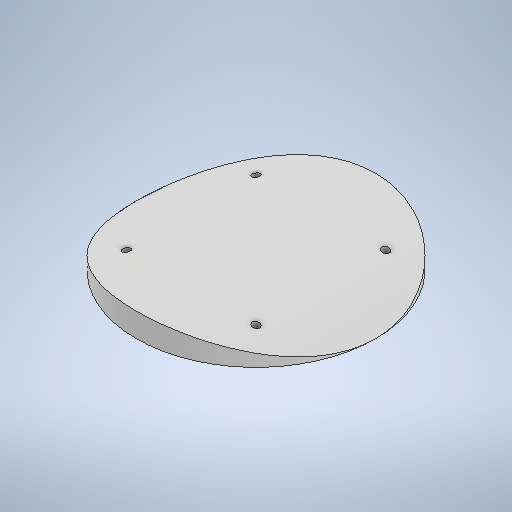
# Autodesk Inventor part: TopHead
Saved by Autodesk Inventor 2025 (Build 290162000, 162)
## iProperties
Created: 2025-09-02
Part Number: TopHead
Material: Generic
Document SubType Name: Modeling
Designer: wangb
Density: 1 g/cm^3
Appearance: Default
Author: wangb
Autodesk Inventor part; units mm, degrees
ref_plane "YZ Plane" through (0, 0, 0) normal (1, 0, 0) x (0, 1, 0)
ref_plane "XZ Plane" through (0, 0, 0) normal (0, 1, 0) x (-1, 0, 0)
ref_plane "XY Plane" through (0, 0, 0) normal (0, 0, 1) x (1, 0, 0)
sketch "Sketch1" plane through (0, 0, 0) normal (0, 0, 1) x (1, 0, 0)
  arc A0 (76.5789, 0) -> (-8.4211, 0) centre (34.0789, -102.0754) ccw
  line L0 (-8.4211, 0) -> (76.5789, 0)
  point P0 (0, 0)
  dimension "d0" = 85
  constraints: 2 end point, 2 point on circle, 1 centre point, 1 horizontal
  measures "d0" distance of L0.start L0.end
extrude "Extrusion1" add sketch "Sketch1" along normal blind 85
sketch "Sketch2" plane through (-8.4211, 0, 0) normal (0, -1, 0) x (1, 0, 0)
  circle A0 centre (7.5, 77.5) radius 0.75
  circle A1 centre (7.5, 7.5) radius 0.75
  circle A2 centre (77.5, 77.5) radius 0.75
  circle A3 centre (77.5, 7.5) radius 0.75
  line L0 (0, 85) -> (85, 85) projected
  line L1 (0, 0) -> (85, 0) projected
  line L2 (85, 0) -> (85, 85) projected
  point P0 (8.4211, 0)
  point P1 (36.7967, 13.095)
  dimension "d3" = 1.5
  dimension "d4" = 1.5
  dimension "d5" = 1.5
  dimension "d6" = 1.5
  dimension "d7" = 70
  dimension "d8" = 7.5
  dimension "d9" = 7.5
  dimension "d10" = 70
  dimension "d11" = 70
  dimension "d12" = 70
  dimension "d13" = 7.5
  dimension "d14" = 7.5
  constraints: 4 centre point
  measures "d3" diameter of A0
  measures "d4" diameter of A1
  measures "d5" diameter of A2
  measures "d6" diameter of A3
  measures "d7" distance of A1.centre A0.centre
  measures "d8" distance from line of L0 A0.centre
  measures "d9" distance from line of L1 A1.centre
  measures "d10" distance of A0.centre A2.centre
  measures "d11" distance of A1.centre A3.centre
  measures "d12" distance of A3.centre A2.centre
  measures "d13" distance from line of L1 A3.centre
  measures "d14" distance from line of L2 A2.centre
extrude "Extrusion2" cut sketch "Sketch2" against normal blind 85
sketch "Sketch3" plane through (-8.4211, 0, 0) normal (0, -1, 0) x (1, 0, 0)
  line L0 (0, 0) -> (0, 85) projected
  line L1 (0, 42.5) -> (85, 42.5)
  line L2 (85, 0) -> (85, 85) projected
  line L3 (0, 85) -> (85, 85) projected
  line L4 (42.5, 85) -> (42.5, 0)
  circle A0 centre (42.5, 42.5) radius 42.5
  line L5 (0, 0) -> (85, 0) projected
  line L6 (85, 85) -> (0, 85)
  line L7 (0, 85) -> (0, 0)
  line L8 (0, 0) -> (85, 0)
  line L9 (85, 0) -> (85, 85)
  point P0 (8.4211, 0)
  dimension "d17" = 42.5
  constraints: 12 end point, 4 midpoint, 2 horizontal, 2 parallel, 1 centre point, 1 perpendicular, 1 tangent, 1 vertical
  measures "d17" distance between parallel lines of L3 L1
extrude "Extrusion3" cut sketch "Sketch3" against normal blind 100 contours L0 A0 L5 | L0 L3 A0 | A0 L2 L5 | L3 L2 A0
sketch "Sketch4" plane through (34.0789, 0, 42.5) normal (0, -1, 0) x (1, 0, 0)
  arc A0 (-42.5, 0) -> (42.5, 0) centre (0, 0) ccw projected
  line L0 (0, 0) -> (42.5, 0) construction
  line L1 (30.052, 30.052) -> (-30.052, 30.052)
  line L2 (-30.052, 30.052) -> (-30.052, -30.052)
  line L3 (-30.052, -30.052) -> (30.052, -30.052)
  line L4 (30.052, -30.052) -> (30.052, 30.052)
  circle A1 centre (-23.052, 23.052) radius 1.3
  circle A2 centre (23.052, 23.052) radius 1.3
  circle A3 centre (-23.052, -23.052) radius 1.3
  circle A4 centre (23.052, -23.052) radius 1.3
  point P0 (-34.0789, -42.5)
  dimension "d21" = 2.6
  dimension "d22" = 2.6
  dimension "d23" = 2.6
  dimension "d24" = 2.6
  dimension "d29" = 7
  dimension "d30" = 7
  dimension "d31" = 7
  dimension "d32" = 7
  dimension "d33" = 7
  dimension "d34" = 7
  dimension "d35" = 7
  dimension "d36" = 7
  constraints: 10 end point, 4 centre point, 3 perpendicular, 3 point on circle, 2 horizontal
  measures "d21" diameter of A1
  measures "d22" diameter of A2
  measures "d23" diameter of A3
  measures "d24" diameter of A4
  measures "d29" distance from line of L1 A1.centre
  measures "d30" distance from line of L4 A4.centre
  measures "d31" distance from line of L4 A2.centre
  measures "d32" distance from line of L3 A3.centre
  measures "d33" distance from line of L2 A3.centre
  measures "d34" distance from line of L2 A1.centre
  measures "d35" distance from line of L1 A2.centre
  measures "d36" distance from line of L3 A4.centre
extrude "Extrusion4" cut sketch "Sketch4" against normal blind 100 contours A1 | A2 | A3 | A4
body "Solid1"
